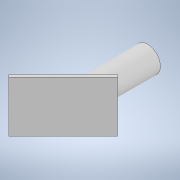
# Autodesk Inventor part: plane cut cylinder
Saved by Autodesk Inventor 2020 (Build 240168000, 168)
## iProperties
Created: 2020-03-04
Part Number: plane cut cylinder
Material: Generic
Document SubType Name: Modeling
Designer: Ethan
Density: 1 g/cm^3
Appearance: Default
Author: Ethan
Autodesk Inventor part; units mm, degrees
ref_plane "YZ Plane" through (0, 0, 0) normal (1, 0, 0) x (0, 1, 0)
ref_plane "XZ Plane" through (0, 0, 0) normal (0, 1, 0) x (-1, 0, 0)
ref_plane "XY Plane" through (0, 0, 0) normal (0, 0, 1) x (1, 0, 0)
sketch "Sketch1" plane through (0, 0, 0) normal (0, 0, 1) x (1, 0, 0)
  circle A0 centre (0, 0) radius 25.4
  dimension "d0" = 50.8
  constraints: 1 centre point, 1 coincident
  measures "d0" diameter of A0
sketch "Sketch1 outline for Extrusion1" plane through (0, 0, 0) normal (0, 0, 1) x (1, 0, 0)
  circle A0 centre (0, 0) radius 25.4
extrude "Extrusion1" add sketch "Sketch1 outline for Extrusion1" against normal blind 127
sketch "Sketch4" plane through (0, 0, 0) normal (0, 0, 1) x (1, 0, 0)
  line L0 (-25.4, -25.4) -> (-25.4, 25.4)
  line L1 (-25.4, 25.4) -> (25.436047, 25.4)
  line L2 (25.436047, 25.4) -> (25.436047, -25.4)
  line L3 (25.436047, -25.4) -> (-25.4, -25.4)
  line L4 (-25.4, -25.4) -> (-25.4, 25.4)
  point P0 (0, 0)
  constraints: 8 end point, 2 parallel, 1 horizontal, 1 perpendicular
sketch "Sketch4 outline for Extrusion3" plane through (0, 0, 0) normal (0, 0, 1) x (1, 0, 0)
  line L0 (-25.4, -25.4) -> (25.436047, -25.4)
  line L1 (-25.4, 25.4) -> (-25.4, -25.4)
  line L2 (25.436047, 25.4) -> (-25.4, 25.4)
  line L3 (25.436047, -25.4) -> (25.436047, 25.4)
extrude "Extrusion3" add sketch "Sketch4 outline for Extrusion3" along normal blind 50.8
chamfer "Chamfer1" distance 50.8 angle 45 1 edges at (25.436, 0, 50.8)
sketch "Sketch5" plane through (-25.4, 0, 0) normal (-1, 0, 0) x (0, 0, 1)
  point P0 (0, 0)
sketch "Sketch6" plane through (0, 0, 0) normal (0, 0, -1) x (-1, 0, 0)
  circle A0 centre (0, 0) radius 25.4
  arc A1 (0, 25.4) -> (-25.4, 0) centre (0, 0) ccw
  line L0 (-25.436047, 25.4) -> (0, 25.4)
  line L1 (-25.4, 0) -> (-25.436047, 25.4)
  line L2 (-25.436047, 25.4) -> (0, 25.4)
  constraints: 4 end point, 4 point on circle, 1 centre point
sketch "Sketch6 outline for Extrusion4" plane through (0, 0, 0) normal (0, 0, -1) x (-1, 0, 0)
  line L0 (-25.436047, 25.4) -> (-25.4, 0)
  line L1 (0, 25.4) -> (-25.436047, 25.4)
  arc A0 (-25.4, 0) -> (0, 25.4) centre (0, 0) cw
extrude "Extrusion4" cut sketch "Sketch6 outline for Extrusion4" against normal blind 50.8
sketch "Sketch7" plane through (0, 0, 0) normal (0, 0, -1) x (-1, 0, 0)
  line L0 (0, 25.4) -> (25.4, 25.4) projected
  line L1 (0, 25.4) -> (25.4, 25.4)
  line L2 (25.4, 25.4) -> (25.4, 0) projected
  line L3 (25.4, 25.4) -> (25.4, 0)
  arc A0 (25.4, 0) -> (0, 25.4) centre (0, 0) ccw
  point P0 (0, 0)
  constraints: 4 end point, 2 collinear, 2 point on circle, 2 tangent, 1 centre point
sketch "Sketch7 outline for Extrusion5" plane through (0, 0, 0) normal (0, 0, -1) x (-1, 0, 0)
  arc A0 (0, 25.4) -> (25.4, 0) centre (0, 0) cw
  line L0 (25.4, 25.4) -> (0, 25.4)
  line L1 (25.4, 0) -> (25.4, 25.4)
extrude "Extrusion5" cut sketch "Sketch7 outline for Extrusion5" against normal blind 50.8
sketch "Sketch8" plane through (0, 0, 0) normal (0, 0, -1) x (-1, 0, 0)
  line L0 (25.4, 0) -> (25.4, -25.4) projected
  line L1 (25.4, 0) -> (25.4, -25.4)
  line L2 (25.4, -25.4) -> (0, -25.4)
  arc A0 (-25.4, 0) -> (0, -25.4) centre (0, 0) ccw projected
  arc A1 (0, -25.4) -> (25.4, 0) centre (0, 0) ccw
  constraints: 4 end point, 2 point on circle, 1 centre point, 1 perpendicular, 1 tangent, 1 vertical
sketch "Sketch8 outline for Extrusion6" plane through (0, 0, 0) normal (0, 0, -1) x (-1, 0, 0)
  arc A0 (25.4, 0) -> (0, -25.4) centre (0, 0) cw
  line L0 (25.4, -25.4) -> (25.4, 0)
  line L1 (0, -25.4) -> (25.4, -25.4)
extrude "Extrusion6" cut sketch "Sketch8 outline for Extrusion6" against normal blind 50.8
sketch "Sketch10" plane through (0, 0, 0) normal (0, 0, -1) x (-1, 0, 0)
  line L0 (-25.4, 0) -> (-25.436047, 25.4)
  line L1 (-25.436047, 25.4) -> (-25.363953, -25.4)
  line L2 (0, -25.4) -> (-25.436047, -25.4)
  line L3 (-25.363953, -25.4) -> (0, -25.4)
  arc A0 (-25.4, 0) -> (0, -25.4) centre (0.036098, 0.036098) ccw
  point P0 (0, 0)
  constraints: 4 end point, 2 collinear, 2 point on circle, 1 centre point, 1 tangent
sketch "Sketch10 outline for Extrusion7" plane through (0, 0, 0) normal (0, 0, -1) x (-1, 0, 0)
  arc A0 (0, -25.4) -> (-25.4, 0) centre (0.036098, 0.036098) cw
  line L0 (-25.363953, -25.4) -> (0, -25.4)
  line L1 (-25.4, 0) -> (-25.363953, -25.4)
extrude "Extrusion7" cut sketch "Sketch10 outline for Extrusion7" against normal blind 50.8
sketch "Sketch11" plane through (-25.363953, -1.352736, 50.8) normal (0.7071068, 0, 0.7071068) x (0.7071068, 0, -0.7071068)
  line L0 (-50.8, -50.8) -> (101.6, -50.8)
  line L1 (101.6, -50.8) -> (101.6, 50.8)
  line L2 (101.6, 50.8) -> (-50.8, 50.8)
  line L3 (-50.8, 50.8) -> (-50.8, -50.8)
  point P0 (53.856048, 1.352736)
  dimension "d18" = 152.4
  dimension "d19" = 101.6
  constraints: 8 end point, 2 parallel, 1 horizontal, 1 perpendicular
  measures "d18" distance of L2.end L1.end
  measures "d19" distance of L1.end L0.end
sketch "Sketch11 outline for Extrusion8" plane through (-25.363953, -1.352736, 50.8) normal (0.7071068, 0, 0.7071068) x (0.7071068, 0, -0.7071068)
  line L0 (101.6, -50.8) -> (101.6, 50.8)
  line L1 (-50.8, -50.8) -> (101.6, -50.8)
  line L2 (-50.8, 50.8) -> (-50.8, -50.8)
  line L3 (101.6, 50.8) -> (-50.8, 50.8)
extrude "Extrusion8" add sketch "Sketch11 outline for Extrusion8" along normal blind 6.35
body "Solid1"
